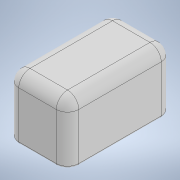
# Autodesk Inventor part: Button_SelectButton
Saved by Autodesk Inventor 2021 (Build 250183000, 183)
## iProperties
Created: 2021-05-07
Part Number: Button_SelectButton
Material: Generic
Document SubType Name: Modeling
Designer: trent
Density: 1 g/cm^3
Appearance: Default
Author: trent
Autodesk Inventor part; units mm, degrees
ref_plane "YZ Plane" through (0, 0, 0) normal (1, 0, 0) x (0, 1, 0)
ref_plane "XZ Plane" through (0, 0, 0) normal (0, 1, 0) x (-1, 0, 0)
ref_plane "XY Plane" through (0, 0, 0) normal (0, 0, 1) x (1, 0, 0)
sketch "Sketch1" plane through (0, 0, 0) normal (0, 1, 0) x (-1, 0, 0)
  line L0 (0, 0) -> (-8, 0)
  line L1 (-8, 0) -> (-8, -14)
  line L2 (-8, -14) -> (0, -14)
  line L3 (0, -14) -> (0, 0)
  dimension "d0" = 8
  dimension "d1" = 14
  constraints: 8 end point, 2 parallel, 1 horizontal, 1 perpendicular
  measures "d0" distance of L1.end L2.end
  measures "d1" distance of L2.end L0.start
extrude "Extrusion1" add sketch "Sketch1" along normal blind 8
fillet "Fillet1" radius 1.5 8 edges at (8, 4, 0) (8, 8, -7) (4, 8, 0) (0, 8, -7) (0, 4, 0) (8, 4, -14) (4, 8, -14) (0, 4, -14)
fillet "Fillet2" radius 0.25 8 edges at (7.5607, 0, -13.5607) (4, 0, -14) (0.4393, 0, -13.5607) (0, 0, -7) (0.4393, 0, -0.4393) (4, 0, 0) (7.5607, 0, -0.4393) (8, 0, -7)
body "Solid1"
